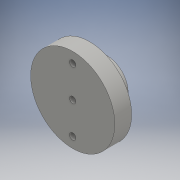
# Autodesk Inventor part: Zoetrope_Motor_Connector
Saved by Autodesk Inventor 2016 (Build 200138000, 138)
## iProperties
Created: 2019-01-08
Part Number: Zoetrope_Motor_Connector
Material: Generic
Document SubType Name: Modeling
Designer: student
Density: 1 g/cm^3
Appearance: Default
Author: student
Autodesk Inventor part; units mm, degrees
ref_plane "YZ Plane" through (0, 0, 0) normal (1, 0, 0) x (0, 1, 0)
ref_plane "XZ Plane" through (0, 0, 0) normal (0, 1, 0) x (-1, 0, 0)
ref_plane "XY Plane" through (0, 0, 0) normal (0, 0, 1) x (1, 0, 0)
sketch "Sketch1" plane through (0, 0, 0) normal (0, 0, 1) x (1, 0, 0)
  line L0 (0, -1.778) -> (4.6736, -1.778) construction
  line L1 (4.6736, -1.778) -> (4.6736, 4.9784) construction
  line L2 (4.6736, 4.9784) -> (0, 4.9784) construction
  line L3 (0, 4.9784) -> (0, -1.778) construction
  line L4 (0, 1.6002) -> (0, 4.0894)
  line L5 (0, 1.6002) -> (0, -0.889)
  line L6 (4.6736, 1.6002) -> (4.6736, 4.0894)
  line L7 (4.6736, 1.6002) -> (4.6736, -0.889)
  arc A0 (4.6736, 4.0894) -> (0, 4.0894) centre (2.3368, 1.4627) ccw
  arc A1 (0, -0.889) -> (4.6736, -0.889) centre (2.3368, 1.7377) ccw
  circle A2 centre (2.3368, 1.6002) radius 6.35
  dimension "d21" = 4.6736
  dimension "d22" = 6.7564
  dimension "d23" = 2.4892
  dimension "d24" = 2.4892
  dimension "d25" = 12.7
  dimension "d30" = 3.5157
  dimension "d31" = 3.5157
  dimension "d32" = 0.2751
  dimension "d33" = 2.3368
  dimension "d34" = 0.1375
  dimension "d35" = 2.3368
  constraints: 16 end point, 4 point on circle, 4 point on line, 3 centre point, 2 midpoint, 2 parallel, 1 horizontal, 1 perpendicular
  measures "d21" distance of L2.end L1.end
  measures "d22" distance of L1.end L0.end
  measures "d23" distance of L4.start L4.end
  measures "d24" distance of L4.start L5.end
  measures "d25" diameter of A2
  measures "d30" radius of A0
  measures "d31" radius of A1
  measures "d32" distance of A1.centre A0.centre
  measures "d33" distance from line of L1 A2.centre
  measures "d34" distance of A0.centre A2.centre
  measures "d35" distance from line of L7 A1.centre
extrude "Extrusion1" add sketch "Sketch1" along normal blind 5.334
sketch "Sketch2" plane through (2.3876, 3.4798, 5.334) normal (0, 0, 1) x (1, 0, 0)
  circle A0 centre (0, -1.8796) radius 0.9525
  circle A1 centre (0, -1.8796) radius 12.7
  line L0 (0, 10.8204) -> (0, 4.4702) construction
  circle A2 centre (-0.0508, -1.8796) radius 6.35 projected
  circle A3 centre (0, 7.6453) radius 0.9525
  line L1 (0, -14.5796) -> (0, -8.2294) construction
  circle A4 centre (0, -11.4045) radius 0.9525
  dimension "d26" = 1.905
  dimension "d27" = 25.4
  dimension "d28" = 1.905
  dimension "d29" = 1.905
  constraints: 4 centre point, 4 end point, 4 point on circle, 2 midpoint, 2 vertical, 1 coincident
  measures "d26" diameter of A0
  measures "d27" diameter of A1
  measures "d28" diameter of A3
  measures "d29" diameter of A4
extrude "Extrusion2" add sketch "Sketch2" along normal blind 5.08 contours A1 | A2
ref_plane "Work Plane1" through (2.3876, 3.4798, -50.8) normal (0, 0, -1) x (-1, 0, 0)
sketch "Sketch5" plane through (2.3876, 3.4798, -50.8) normal (0, 0, -1) x (-1, 0, 0)
  line L0 (2.3876, 0.6096) -> (2.3876, -4.3688) projected
  arc A0 (2.3876, 0.6096) -> (-2.286, 0.6096) centre (0.0508, -2.0171) ccw projected
  line L1 (-2.286, -4.3688) -> (-2.286, 0.6096) projected
  arc A1 (-2.286, -4.3688) -> (2.3876, -4.3688) centre (0.0508, -1.7421) ccw projected
  circle A2 centre (0.0508, -1.8796) radius 6.35 projected
  point P0 (2.3876, -3.4798)
body "Solid1"
